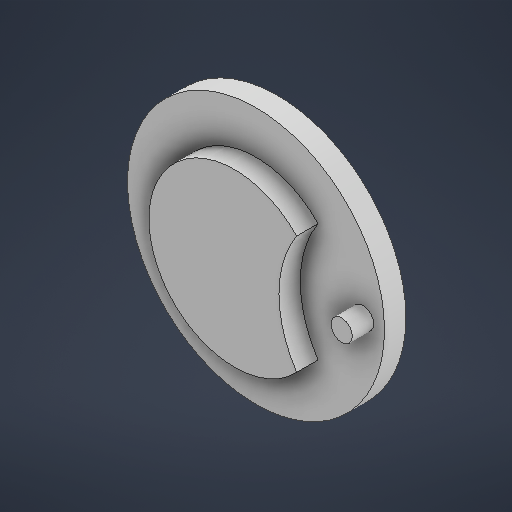
# Autodesk Inventor part: geniva1
Saved by Autodesk Inventor 2026.3 (Build 303398000, 398)
## iProperties
Created: 2026-04-30
Part Number: geniva1
Material: Generic
Document SubType Name: Modeling
Designer: frede
Density: 1 g/cm^3
Appearance: Default
Author: frede
Autodesk Inventor part; units mm, degrees
ref_plane "YZ Plane" through (0, 0, 0) normal (1, 0, 0) x (0, 1, 0)
ref_plane "XZ Plane" through (0, 0, 0) normal (0, 1, 0) x (-1, 0, 0)
ref_plane "XY Plane" through (0, 0, 0) normal (0, 0, 1) x (1, 0, 0)
sketch "Sketch2" plane through (0, 0, 0) normal (0, 0, 1) x (1, 0, 0)
  circle A0 centre (0, 0) radius 30
  dimension "d21" = 60
  constraints: 1 centre point, 1 coincident
  measures "d21" diameter of A0
extrude "Extrusion1" add sketch "Sketch2" along normal blind 5
sketch "Sketch4" plane through (0, 0, 5) normal (0, 0, 1) x (1, 0, 0)
  circle A0 centre (0, 0) radius 20
  circle A1 centre (25, 0) radius 2.5
  circle A2 centre (35.36, 0) radius 25
  point P0 (14.4984, -13.7766)
  point P1 (14.4984, 13.7766)
  dimension "d36" = 40
  dimension "d37" = 5
  dimension "d39" = 50
  dimension "d42" = 35.36
  constraints: 3 centre point, 1 coincident
  measures "d36" diameter of A0
  measures "d37" diameter of A1
  measures "d39" diameter of A2
  measures "d42" distance of point (0, 0) A2.centre
extrude "Extrusion3" add sketch "Sketch4" along normal blind 5 contours A2 A0 | A1 picked at (0.3534, 0)
body "Solid1"
